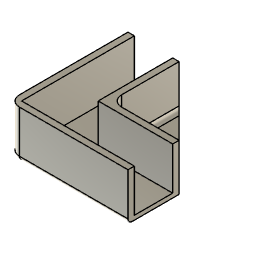
Angle Assembly Template (Autodesk Fusion 360 design; units mm, degrees)
Autodesk Fusion 360 part; units mm, degrees
sketch "Sketch1" plane through (0, 0, 0) normal (0, 0, 1) x (1, 0, 0)
  line L0 (0, 0) -> (18, 0) construction
  line L1 (18, 18) -> (18, 50)
  line L2 (0, 50) -> (0, 0)
  line L3 (0, 0) -> (50, 0)
  line L4 (50, 18) -> (18, 18)
  line L5 (0, 18) -> (0, 0) construction
  line L6 (53, 21) -> (21, 21)
  line L7 (21, 21) -> (21, 53)
  line L8 (-3, 53) -> (-3, -3)
  line L9 (-3, -3) -> (53, -3)
  line L10 (50, 18) -> (53, 18)
  line L11 (50, 0) -> (53, 0)
  line L12 (0, 50) -> (0, 53)
  line L13 (18, 50) -> (18, 53)
  line L14 (21, 53) -> (18, 53)
  line L15 (0, 53) -> (-3, 53)
  line L16 (53, -3) -> (53, 0)
  line L17 (53, 18) -> (53, 21)
  dimension "d1" = 18
  dimension "d2" = 50
  dimension "d3" = 50
  dimension "d4" = 18
  constraint horizontal L0
  constraint vertical L1
  constraint vertical L2
  constraint coincident L0.start L2.end
  constraint horizontal L3
  constraint horizontal L4
  constraint vertical L5
  constraint coincident L10.end L16
  constraint perpendicular L10 L16
  constraint perpendicular L11 L16
  constraint coincident L12.end L14
  constraint perpendicular L12 L14
  constraint perpendicular L13 L14
  constraint collinear L14 L15
  constraint collinear L16 L17
  measures "d1" distance of L0.start L0.end
  measures "d2" distance of L0.start L2.start
  measures "d3" distance of L0.start L3.end
  measures "d4" distance of L0.start L5.start
extrude "Extrude1" add sketch "Sketch1" along normal blind 20 makes body 1 at (18, 29.6667, 13.3333) makes body 2 at (15.6667, -3, 6.6667)
sketch "Sketch2" plane through (0, 0, 0) normal (0, 0, -1) x (1, 0, 0)
  line L0 (53, -18) -> (18, -18)
  line L1 (18, -18) -> (18, -53)
  line L2 (18, -53) -> (21, -53)
  line L3 (21, -53) -> (21, -21)
  line L4 (21, -21) -> (53, -21)
  line L5 (53, -21) -> (53, -18)
  line L6 (0, -53) -> (0, 0)
  line L7 (0, 0) -> (53, 0)
  line L8 (53, 0) -> (53, 3)
  line L9 (53, 3) -> (-3, 3)
  line L10 (-3, 3) -> (-3, -53)
  line L11 (-3, -53) -> (0, -53)
  line L12 (-3, 3) -> (53, 3) construction
  line L13 (53, 3) -> (53, -21)
  line L14 (53, -21) -> (21, -53)
  line L15 (21, -53) -> (-3, -53)
  line L16 (-3, -53) -> (-3, 3)
  line L17 (-3, 3) -> (53, 3)
  constraint coincident L9.end L10.start
  constraint coincident L8.end L9.start
  constraint coincident L4.end L5.start
  constraint coincident L2.end L3.start
  constraint coincident L10.end L11.start
extrude "Extrude2" add sketch "Sketch2" along normal blind 2 bodies 1 2
fillet "Fillet1" radius 5 2 edges at (21, 21, 10) (-3, -3, 9) on bodies 1
fillet "Fillet2" radius 2 6 edges at (27.5, -3, -2) (-1.5355, -1.5355, -2) (-3, 27.5, -2) (39.5, 21, 0) (22.4645, 22.4645, 0) (21, 39.5, 0) on bodies 1
